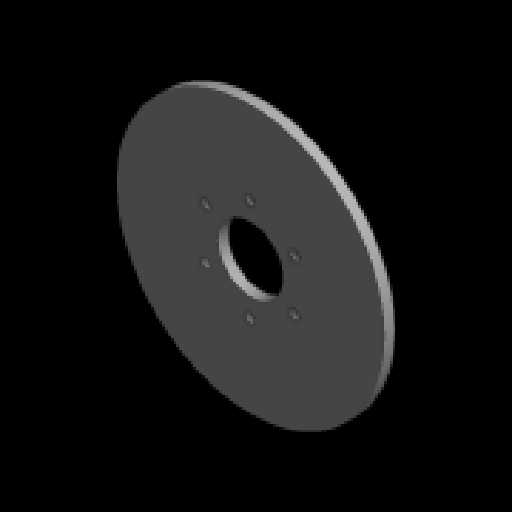
# Autodesk Inventor part: NeckBase
Saved by Autodesk Inventor 2025.2 (Build 292293000, 293)
## iProperties
Created: 2025-08-15
Part Number: NeckBase
Material: Generic
Document SubType Name: Sheet Metal
Designer: valer
Density: 1 g/cm^3
Sheet Metal Rule: Default
Appearance: Default
Author: valer
Autodesk Inventor part; units mm, degrees
ref_plane "YZ Plane" through (0, 0, 0) normal (1, 0, 0) x (0, 1, 0)
ref_plane "XZ Plane" through (0, 0, 0) normal (0, 1, 0) x (-1, 0, 0)
ref_plane "XY Plane" through (0, 0, 0) normal (0, 0, 1) x (1, 0, 0)
sketch "Base" plane through (0, 0, 0) normal (0, 0, 1) x (1, 0, 0)
  circle A0 centre (0, 7.375) radius 56.125 construction
  line L0 (0, -79.425) -> (0, 94.175) construction
  circle A1 centre (0, 7.375) radius 62
  line L1 (-34.5, -17.2623) -> (-48.798, -11.1931) construction
  point P0 (0, 0)
  point P1 (0, -28.5)
  dimension "d1" = 124
  dimension "d39" = 5.875
  measures "d1" diameter of A1
  measures "d39" radial gap between concentric circles of A0 A1
extrude "Plate1" add sketch "Base" along normal blind 5
sketch "HubCenterHole" plane through (0, 7.375, 5) normal (0, 0, 1) x (1, 0, 0)
  circle A0 centre (0, 0) radius 15 construction
  circle A1 centre (0, 0) radius 15.25
  point P0 (0, -7.375)
  dimension "d79" = 0.25
  constraints: 1 centre point, 1 coincident
  measures "d79" radial gap between concentric circles of A1 A0
extrude "HubCenterHoleFeature" cut sketch "HubCenterHole" against normal blind 5
sketch "HubMountHoles" plane through (0, 7.375, 5) normal (0, 0, 1) x (1, 0, 0)
  circle A0 centre (0, -23.75) radius 2.5 construction
  circle A1 centre (-20.5681, -11.875) radius 2.5 construction
  circle A2 centre (-20.5681, 11.875) radius 2.5 construction
  circle A3 centre (0, 23.75) radius 2.5 construction
  circle A4 centre (20.5681, 11.875) radius 2.5 construction
  circle A5 centre (20.5681, -11.875) radius 2.5 construction
  circle A6 centre (0, -23.75) radius 2.5 construction
  circle A7 centre (0, -23.75) radius 2.2
  circle A8 centre (20.5681, -11.875) radius 2.2
  circle A9 centre (20.5681, 11.875) radius 2.2
  circle A10 centre (0, 23.75) radius 2.2
  circle A11 centre (-20.5681, -11.875) radius 2.2
  circle A12 centre (-20.5681, 11.875) radius 2.2
  point P0 (0, -7.375)
extrude "HubMountHolesFeature" cut sketch "HubMountHoles" against normal blind 5
sketch "BracketMountHoles" plane through (0, 7.375, 5) normal (0, 0, 1) x (1, 0, 0)
  circle A0 centre (-35, -19.4802) radius 2 construction
  circle A1 centre (35, -19.4802) radius 2 construction
  circle A2 centre (-35, 22.9931) radius 2 construction
  circle A3 centre (-35, -19.4802) radius 2 construction
  arc A4 (-56, -19.7436) -> (-50, -25.7436) centre (-50, -19.7436) ccw construction
  line L0 (-22, -25.7436) -> (-50, -25.7436) construction
  line L1 (-22, -25.7436) -> (-22, 29.2564) construction
  line L2 (-50, 29.2564) -> (-22, 29.2564) construction
  arc A5 (-50, 29.2564) -> (-56, 23.2564) centre (-50, 23.2564) ccw construction
  line L3 (-56, -19.7436) -> (-56, 23.2564) construction
  circle A6 centre (35, 22.9931) radius 2 construction
  circle A7 centre (35, -19.4802) radius 2 construction
  arc A8 (50, -25.7436) -> (56, -19.7436) centre (50, -19.7436) ccw construction
  line L4 (56, -19.7436) -> (56, 23.2564) construction
  arc A9 (56, 23.2564) -> (50, 29.2564) centre (50, 23.2564) ccw construction
  line L5 (50, 29.2564) -> (22, 29.2564) construction
  line L6 (22, -25.7436) -> (22, 29.2564) construction
  line L7 (22, -25.7436) -> (50, -25.7436) construction
  circle A10 centre (-35, -19.4802) radius 1.7
  circle A11 centre (-35, 22.9931) radius 1.7
  circle A12 centre (35, -19.4802) radius 1.7
  circle A13 centre (35, 22.9931) radius 1.7
  point P0 (0, -7.375)
  dimension "d88" = 4
  dimension "d89" = 3.4
  dimension "d90" = 3.4
  dimension "d91" = 3.4
  dimension "d92" = 3.4
  constraints: 4 centre point, 4 coincident
  measures "d88" diameter of A0
  measures "d89" diameter of A10
  measures "d90" diameter of A11
  measures "d91" diameter of A12
  measures "d92" diameter of A13
extrude "BracketMountHolesFeature" cut sketch "BracketMountHoles" against normal blind 5
equation "\"d12\" = Thickness"
equation "\"BendRadius\" = Thickness"
equation "\"BendReliefWidth\" = Thickness"
equation "\"BendReliefDepth\" = 0.5 * Thickness"
equation "\"TransitionRadius\" = BendRadius"
equation "\"JacobiRadiusSize\" = BendRadius"
equation "\"GapSize\" = Thickness"
equation "\"Thickness\" = 5"
body "Solid1"
